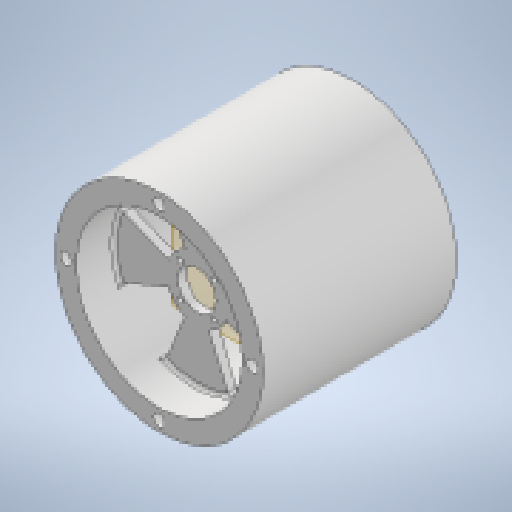
# Autodesk Inventor part: j1 mount
Saved by Autodesk Inventor 2025 (Build 290162000, 162)
## iProperties
Created: 2025-07-04
Part Number: j1 mount
Material: 一般
Document SubType Name: Modeling
Designer: gavin
Density: 1 g/cm^3
Appearance: 預設
Author: gavin
Autodesk Inventor part; units mm, degrees
ref_plane "YZ Plane" through (0, 0, 0) normal (1, 0, 0) x (0, 1, 0)
ref_plane "XZ Plane" through (0, 0, 0) normal (0, 1, 0) x (-1, 0, 0)
ref_plane "XY Plane" through (0, 0, 0) normal (0, 0, 1) x (1, 0, 0)
sketch "草圖1" plane through (0, 0, 0) normal (0, 0, 1) x (1, 0, 0)
  circle A0 centre (0, 0) radius 60
  circle A1 centre (0, 0) radius 48
  dimension "d0" = 120
  dimension "d1" = 96
  constraints: 2 centre point, 2 coincident
  measures "d0" diameter of A0
  measures "d1" diameter of A1
extrude "擠出1" add sketch "草圖1" along normal blind 27 and the other way blind 85
sketch "草圖2" plane through (0, 0, 27) normal (0, 0, 1) x (1, 0, 0)
  circle A0 centre (0, 0) radius 54 construction
  circle A1 centre (0, -54) radius 3.3
  circle A2 centre (54, 0) radius 3.3
  circle A3 centre (0, 54) radius 3.3
  circle A4 centre (-54, 0) radius 3.3
  dimension "d6" = 108
  dimension "d7" = 6.6
  dimension "d10" = 360
  constraints: 4 centre point, 1 coincident, 1 vertical alignment, 11 other
  measures "d7" diameter of A1
extrude "擠出2" cut sketch "草圖2" against normal blind 20
ref_plane "工作平面1" through (0, 0, 0) normal (0, 0, 1) x (1, 0, 0)
sketch "草圖3" plane through (0, 0, 0) normal (0, 0, 1) x (1, 0, 0)
  circle A0 centre (0, 0) radius 11
  circle A1 centre (-9.899495, -9.899495) radius 1.5
  circle A2 centre (9.899495, -9.899495) radius 1.5
  circle A3 centre (-9.899495, 9.899495) radius 1.5
  circle A4 centre (9.899495, 9.899495) radius 1.5
  circle A5 centre (0, 0) radius 18
  circle A6 centre (0, 0) radius 48
  line L0 (0, -18) -> (0, -48) construction
  line L1 (6.888302, -16.629832) -> (18.368805, -44.346218)
  line L2 (-6.888302, -16.629832) -> (-18.368805, -44.346218)
  line L3 (18, 0) -> (48, 0) construction
  line L4 (16.629832, 6.888302) -> (44.346218, 18.368805)
  line L5 (16.629832, -6.888302) -> (44.346218, -18.368805)
  line L6 (0, 18) -> (0, 48) construction
  line L7 (-6.888302, 16.629832) -> (-18.368805, 44.346218)
  line L8 (6.888302, 16.629832) -> (18.368805, 44.346218)
  line L9 (-18, 0) -> (-48, 0) construction
  line L10 (-16.629832, -6.888302) -> (-44.346218, -18.368805)
  line L11 (-16.629832, 6.888302) -> (-44.346218, 18.368805)
  circle A7 centre (0, 0) radius 11.1
  circle A8 centre (-9.899495, -9.899495) radius 1.7
  circle A9 centre (9.899495, -9.899495) radius 1.7
  circle A10 centre (9.899495, 9.899495) radius 1.7
  circle A11 centre (-9.899495, 9.899495) radius 1.7
  point P0 (-18.368805, -44.346218)
  dimension "d17" = 360
  dimension "d22" = 0.1
  dimension "d23" = 0.2
  dimension "d26" = 360
  constraints: 24 end point, 5 centre point, 5 point on circle, 1 symmetric about line, 1 vertical, 46 other
  measures "d22" radial gap between concentric circles of A0 A7
  measures "d23" radial gap between concentric circles of A1 A8
extrude "擠出3" add sketch "草圖3" along normal blind 5 contours A5 | A5 L4 A6 L5 | A5 L7 A6 L8 | L1 A6 L2 A5 | A5 L10 A6 L11
fillet "圓角1" radius 2 18 edges at (47.0777, 9.3643, 5) (47.0777, -9.3643, 5) (0, -48, 5) (-18.3688, -44.3462, 2.5) (18.3688, -44.3462, 2.5) (-48, 0, 5) (44.3462, 18.3688, 2.5) (44.3462, -18.3688, 2.5) (0, 48, 5) (18.3688, 44.3462, 2.5) (-18.3688, 44.3462, 2.5) (0, 48, 0) (-48, 0, 0) (-44.3462, 18.3688, 2.5) (0, -48, 0) (47.0777, -9.3643, 0) (47.0777, 9.3643, 0) (-44.3462, -18.3688, 2.5)
